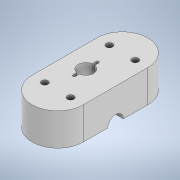
# Autodesk Inventor part: Podstawka_najwieksza_os
Saved by Autodesk Inventor 2020 (Build 240168000, 168)
## iProperties
Created: 2021-03-05
Part Number: Podstawka_najwieksza_os
Material: Generic
Document SubType Name: Modeling
Designer: patry
Density: 1 g/cm^3
Appearance: Default
Author: patry
Autodesk Inventor part; units mm, degrees
ref_plane "YZ Plane" through (0, 0, 0) normal (1, 0, 0) x (0, 1, 0)
ref_plane "XZ Plane" through (0, 0, 0) normal (0, 1, 0) x (-1, 0, 0)
ref_plane "XY Plane" through (0, 0, 0) normal (0, 0, 1) x (1, 0, 0)
sketch "Sketch1" plane through (0, 0, 0) normal (0, 1, 0) x (-1, 0, 0)
  circle A0 centre (-21.8, -50) radius 6.025
  circle A1 centre (-25, -75) radius 19.8
  circle A2 centre (-25, -25) radius 19.8
  line L0 (-5.2, -75) -> (-5.2, -25)
  line L1 (-44.8, -75) -> (-44.8, -25)
  line L2 (-21.8, -50) -> (-22.8, -50)
  line L3 (-22.8, -50) -> (-22.8, -60)
  line L4 (-22.8, -60) -> (-21.8, -60)
  line L5 (-21.8, -60) -> (-21.8, -50)
  line L6 (-22.8, -60) -> (-20.8, -60)
  line L7 (-20.8, -60) -> (-20.8, -40)
  line L8 (-20.8, -40) -> (-22.8, -40)
  line L9 (-22.8, -40) -> (-22.8, -60)
  point P0 (0, 0)
  point P1 (0, 0)
  point P2 (47, 5)
  point P3 (47, 93)
  point P4 (47, 95)
  point P5 (47, 25)
  point P6 (45, 25)
  point P7 (45, 75)
  point P8 (47, 75)
  point P9 (25, 5)
  point P10 (45, 25)
  point P11 (25, 95)
  point P12 (45, 75)
  point P13 (-22.8, -44.0586)
  point P14 (-20.8, -44.0586)
  point P15 (-20.8, -55.9414)
  point P16 (-22.8, -55.9414)
  dimension "d7" = 12.05
  dimension "d10" = 39.6
  dimension "d11" = 39.6
  dimension "d12" = 1
  dimension "d13" = 10
  dimension "d14" = 2
  dimension "d15" = 20
  constraints: 20 end point, 4 parallel, 4 point on circle, 3 centre point, 2 horizontal, 2 perpendicular, 2 tangent
  measures "d7" diameter of A0
  measures "d10" diameter of A1
  measures "d11" diameter of A2
  measures "d12" distance of L4.end L3.end
  measures "d13" distance of L3.end L2.end
  measures "d14" distance of L8.end L7.end
  measures "d15" distance of L7.end L6.end
extrude "Extrusion1" add sketch "Sketch1" along normal blind 25 contours A0 A2 L0 A1 | A0 L7 L8 L9 A2 | A1 A0 L3 L4 L6 L7 | A2 A0 A1 L1
sketch "Sketch2" plane through (0, 0, 0) normal (0, -1, 0) x (1, 0, 0)
  arc A0 (22.8, -55.9414) -> (22.8, -44.0586) centre (21.8, -50) ccw projected
  circle A1 centre (21.8, -50) radius 6.025
  line L0 (21.8, -50) -> (44.8, -50)
  line L1 (44.8, -25) -> (44.8, -75) projected
  line L2 (44.8, -50) -> (21.8, -50)
  line L3 (21.8, -50) -> (21.8, -56.025)
  line L4 (21.8, -56.025) -> (44.8, -56.025)
  line L5 (44.8, -56.025) -> (44.8, -50)
  line L6 (44.8, -50) -> (21.8, -50)
  line L7 (21.8, -50) -> (21.8, -43.975)
  line L8 (21.8, -43.975) -> (44.8, -43.975)
  line L9 (44.8, -43.975) -> (44.8, -50)
  point P0 (0, 0)
  constraints: 18 end point, 4 parallel, 3 point on circle, 2 horizontal, 2 perpendicular, 1 centre point, 1 coincident, 1 midpoint
extrude "Extrusion2" cut sketch "Sketch2" against normal blind 6 contours A0 L0 L1 L4 A1 | A0 A1 L8 L1 L0
fillet "Fillet1" radius 6 2 edges at (33.8, 6, -56.025) (33.8, 6, -43.975)
fillet "Fillet2" radius 6 3 edges at (27.825, 6, -50) (25.8525, 4.0429, -45.5416) (25.8524, 4.0428, -54.4585)
fillet "Fillet3" radius 1 4 edges at (20.8, 12.5, -40) (22.8, 12.5, -40) (20.8, 12.5, -60) (22.8, 12.5, -60)
sketch "Sketch4" plane through (0, 0, 0) normal (0, -1, 0) x (1, 0, 0)
  circle A0 centre (21.8, -50) radius 6.025
  circle A1 centre (25, -75) radius 19.8
  circle A2 centre (25, -25) radius 19.8
  line L0 (5.2, -75) -> (5.2, -25)
  line L1 (44.8, -75) -> (44.8, -25)
  line L2 (21.8, -50) -> (22.8, -50)
  line L3 (22.8, -50) -> (22.8, -60)
  line L4 (22.8, -60) -> (21.8, -60)
  line L5 (21.8, -60) -> (21.8, -50)
  line L6 (22.8, -60) -> (20.8, -60)
  line L7 (20.8, -60) -> (20.8, -40)
  line L8 (20.8, -40) -> (22.8, -40)
  line L9 (22.8, -40) -> (22.8, -60)
  line L10 (25, -25) -> (35, -25)
  line L11 (35, -25) -> (35, -26)
  line L12 (35, -26) -> (25, -26)
  line L13 (25, -26) -> (25, -25)
  line L14 (35, -25) -> (15, -25)
  line L15 (15, -25) -> (15, -75)
  line L16 (15, -75) -> (35, -75)
  line L17 (35, -75) -> (35, -25)
  point P0 (47, 5)
  point P1 (47, 93)
  point P2 (47, 95)
  point P3 (47, 25)
  point P4 (45, 25)
  point P5 (45, 75)
  point P6 (47, 75)
  point P7 (25, 5)
  point P8 (45, 25)
  point P9 (25, 95)
  point P10 (45, 75)
  point P11 (-22.8, -44.0586)
  point P12 (-20.8, -44.0586)
  point P13 (-20.8, -55.9414)
  point P14 (-21.8, -60)
  point P15 (-22.8, -55.9414)
  dimension "d30" = 10
  dimension "d31" = 1
  dimension "d32" = 20
  dimension "d33" = 50
  constraints: 36 end point, 4 parallel, 4 point on circle, 3 centre point, 2 horizontal, 2 perpendicular
  measures "d30" distance of L11.end L12.end
  measures "d31" distance of L10.end L11.end
  measures "d32" distance of L16.end L15.end
  measures "d33" distance of L15.end L14.end
hole "Hole1" at (35, 0, -25) at (15, 0, -25) at (15, 0, -75) at (35, 0, -75) direction (0, 1, 0) diameter 5 end through all counterbore diameter 8.4 counterbore depth 5
body "Solid1"
